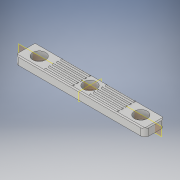
# Autodesk Inventor part: x_carriage_aio_clamp
Saved by Autodesk Inventor 2019 (Build 230136000, 136)
## iProperties
Created: 2019-09-15
Part Number: x_carriage_aio_clamp
Material: Generisch
Document SubType Name: Modeling
Designer: marc
Density: 1 g/cm^3
Appearance: Vorgabe
Author: marc
## iProperties of the stored document x_carriage_aio_clamp_3D-Druck.ipt
Created: 2019-09-15
Part Number: x_carriage_aio_clamp_3D-Druck
Material: Generisch
Document SubType Name: Modeling
Designer: marc
Density: 1 g/cm^3
Appearance: Vorgabe
Author: marc
Autodesk Inventor part; units mm, degrees
ref_plane "YZ Plane" through (0, 0, 0) normal (1, 0, 0) x (0, 1, 0)
ref_plane "XZ Plane" through (0, 0, 0) normal (0, 1, 0) x (-1, 0, 0)
ref_plane "XY Plane" through (0, 0, 0) normal (0, 0, 1) x (1, 0, 0)
sketch "Skizze1" plane through (0, 0, 0) normal (0, 1, 0) x (-1, 0, 0)
  line L0 (0, 0) -> (32, 0)
  line L1 (32, 0) -> (32, 5)
  line L2 (32, 5) -> (0, 5)
  line L3 (0, 5) -> (0, 0)
  dimension "d0" = 32
  dimension "d1" = 5
  constraints: 8 end point, 2 parallel, 1 horizontal, 1 perpendicular
  measures "d0" distance of L0.start L0.end
  measures "d1" distance of L2.end L0.start
extrude "Extrusion1" add sketch "Skizze1" along normal blind 2
ref_plane "Arbeitsebene1" through (-32, 0, 2.5) normal (0, 0, 1) x (1, 0, 0)
ref_plane "Arbeitsebene2" through (-16, 0, 5) normal (1, 0, 0) x (0, 0, -1)
sketch "Skizze2" plane through (0, 2, 0) normal (0, 1, 0) x (1, 0, 0)
  line L0 (6.4, -2.5) -> (-38.4, -2.5) projected
  line L1 (-16, 1) -> (-16, -6) projected
  point P0 (0, 0)
  point P1 (-28.5, -2.5)
  point P2 (-16, -2.5)
  point P3 (-3.5, -2.5)
  dimension "d4" = 25
  dimension "d5" = 12.5
  constraints: 2 horizontal alignment, 1 midpoint, 1 point on line
  measures "d4" distance of point (-28.5, -2.5) point (-3.5, -2.5)
  measures "d5" distance of point (-28.5, -2.5) point (-16, -2.5)
hole "Bohrung1" at (-28.5, 2, 2.5) at (-16, 2, 2.5) at (-3.5, 2, 2.5) direction (0, -1, 0) diameter 3.2 end through all
sketch "Skizze3" plane through (0, 2, 0) normal (0, 1, 0) x (1, 0, 0)
  line L0 (-18, -4.75) -> (-25, -4.75)
  line L1 (-25, -4.75) -> (-25, -4.25)
  line L2 (-25, -4.25) -> (-18, -4.25)
  line L3 (-18, -4.25) -> (-18, -4.75)
  line L4 (-18, -3.75) -> (-25, -3.75)
  line L5 (-25, -3.75) -> (-25, -3.25)
  line L6 (-25, -3.25) -> (-18, -3.25)
  line L7 (-18, -3.25) -> (-18, -3.75)
  line L8 (-18, -2.75) -> (-25, -2.75)
  line L9 (-25, -2.75) -> (-25, -2.25)
  line L10 (-25, -2.25) -> (-18, -2.25)
  line L11 (-18, -2.25) -> (-18, -2.75)
  line L12 (-18, -1.75) -> (-25, -1.75)
  line L13 (-25, -1.75) -> (-25, -1.25)
  line L14 (-25, -1.25) -> (-18, -1.25)
  line L15 (-18, -1.25) -> (-18, -1.75)
  line L16 (-18, -0.75) -> (-25, -0.75)
  line L17 (-25, -0.75) -> (-25, -0.25)
  line L18 (-25, -0.25) -> (-18, -0.25)
  line L19 (-18, -0.25) -> (-18, -0.75)
  line L20 (-16, 1) -> (-16, -6) projected
  line L21 (-32, -5) -> (0, -5) projected
  line L22 (0, 0) -> (-32, 0) projected
  dimension "d13" = 2
  dimension "d14" = 7
  dimension "d15" = 0.5
  dimension "d16" = 0.5
  dimension "d17" = 0.5
  dimension "d18" = 0.5
  dimension "d19" = 0.5
  dimension "d20" = 0.25
  dimension "d21" = 0.25
  constraints: 40 end point, 10 parallel, 5 horizontal, 5 perpendicular, 5 point on line, 4 collinear, 3 vertical alignment
  measures "d13" distance between parallel lines of L3 L20
  measures "d14" distance of L0.start L0.end
  measures "d15" distance of L0.end L1.end
  measures "d16" distance of L4.end L1.end
  measures "d17" distance of L8.end L5.end
  measures "d18" distance of L9.end L12.end
  measures "d19" distance of L16.end L13.end
  measures "d20" distance between parallel lines of L21 L0
  measures "d21" distance from line of L22 L17.end
extrude "Extrusion2" add sketch "Skizze3" along normal blind 0.2
fillet "Rundung1" radius 0.25 10 edges at (-21.5, 2.2, 4.25) (-21.5, 2.2, 4.75) (-21.5, 2.2, 3.75) (-21.5, 2.2, 3.25) (-21.5, 2.2, 2.75) (-21.5, 2.2, 2.25) (-21.5, 2.2, 1.75) (-21.5, 2.2, 1.25) (-21.5, 2.2, 0.75) (-21.5, 2.2, 0.25)
mirror "Spiegeln1" about plane through (-16, 0, 5) normal (1, 0, 0) of "Rundung1", "Extrusion2"
chamfer "Fase1" distance 0.25 angle 45 4 edges at (-16, 2, 5) (-16, 2, 0) (0, 2, 2.5) (-32, 2, 2.5)
fillet "Rundung2" radius 1 4 edges at (-32, 0.875, 5) (-32, 0.875, 0) (0, 0.875, 5) (0, 0.875, 0)
equation "\"d5\" = 0.5 * d4"
equation "\"d16\" = d15"
equation "\"d17\" = d16"
equation "\"d18\" = d17"
equation "\"d19\" = d17"
